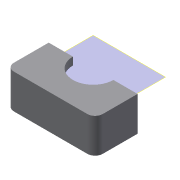
# Autodesk Inventor part: 20_Cube_Insert_Syringepump_Micro_syringeclamp_v3
Saved by Autodesk Inventor 2022 (Build 260153000, 153)
## iProperties
Created: 2022-01-11
Part Number: 20_Cube_Insert_Syringepump_Micro_syringeclamp_v3
Material: Generisch
Document SubType Name: Modeling
Designer: diederichbenedict
Density: 1 g/cm^3
Appearance: Vorgabe
Author: diederichbenedict
Autodesk Inventor part; units mm, degrees
ref_plane "YZ Plane" through (0, 0, 0) normal (1, 0, 0) x (0, 1, 0)
ref_plane "XZ Plane" through (0, 0, 0) normal (0, 1, 0) x (-1, 0, 0)
ref_plane "XY Plane" through (0, 0, 0) normal (0, 0, 1) x (1, 0, 0)
ref_plane "Arbeitsebene1" through (-12.85, 3.6, -4.5) normal (0, -1, 0) x (0, 0, 1)
sketch "Skizze1" plane through (-12.85, 3.6, -4.5) normal (0, -1, 0) x (0, 0, 1)
  circle A0 centre (0, 0) radius 4.3 construction
  line L0 (0.4805, 5.7801) -> (0.4805, 4.5246)
  line L1 (0.4805, -4.5246) -> (0.4805, -5.7801)
  line L2 (0, -5.8) -> (5.55, -5.8)
  line L3 (5.55, -5.8) -> (5.55, 5.8)
  line L4 (5.55, 5.8) -> (0, 5.8)
  line L5 (0, 5.8) -> (0, -5.8)
  line L6 (0, -4.55) -> (4.55, -4.55)
  line L7 (4.55, -4.55) -> (4.55, 4.55)
  line L8 (4.55, 4.55) -> (0, 4.55)
  line L9 (0, 4.55) -> (0, -4.55)
  point P0 (4.5, -12.85)
  point P1 (0, 4.55)
  dimension "d2" = 0
  dimension "d27" = 0
  dimension "d28" = 1
  constraints: 20 end point, 4 parallel, 2 horizontal, 2 perpendicular, 2 vertical, 1 point on line
  measures "d2" distance between parallel lines of L1 L0
  measures "d27" distance from line of A0.centre L5
  measures "d28" distance between parallel lines of L7 L3
extrude "Extrusion1" add sketch "Skizze1" along normal blind 2.5 contours L5 L6 L7 L8 L4 L3 L2
sketch "Skizze2" plane through (-12.85, 1.1, -4.5) normal (0, -1, 0) x (1, 0, 0)
  line L0 (-5.7801, 0.4805) -> (5.7801, 0.4805)
  line L1 (-5.8, 0) -> (-4.55, 0) projected
  line L2 (-4.55, 0) -> (-4.55, 4.55) projected
  line L3 (-4.55, 4.55) -> (4.55, 4.55) projected
  line L4 (4.55, 4.55) -> (4.55, 0) projected
  line L5 (4.55, 0) -> (5.8, 0) projected
  line L6 (5.8, 0) -> (5.8, 5.55) projected
  line L7 (5.8, 5.55) -> (-5.8, 5.55) projected
  line L8 (-5.8, 5.55) -> (-5.8, 0) projected
  line L9 (-4.55, 0) -> (4.55, 0)
  point P0 (12.85, 4.5)
  constraints: 4 end point, 2 horizontal
extrude "Extrusion2" add sketch "Skizze2" along normal blind 1
sketch "Skizze7" plane through (-12.85, 3.6, -4.5) normal (0, 1, 0) x (1, 0, 0)
  line L0 (-5.8, 0) -> (-4.55, 0) projected
  line L1 (-5.8, -5.55) -> (-5.8, 0) projected
  line L2 (5.8, -5.55) -> (-5.8, -5.55) projected
  line L3 (5.8, 0) -> (5.8, -5.55) projected
  line L4 (4.55, 0) -> (5.8, 0) projected
  line L5 (4.55, -4.55) -> (4.55, 0) projected
  line L6 (-4.55, -4.55) -> (4.55, -4.55) projected
  line L7 (-4.55, 0) -> (-4.55, -4.55) projected
  line L8 (4.55, 0) -> (-4.55, 0)
  line L9 (-4.55, -4.55) -> (4.55, -4.55) projected
  circle A0 centre (0, 0) radius 2.6359
  point P0 (12.85, -4.5)
  point P1 (2.6359, 0)
  point P2 (-2.6359, 0)
  constraints: 2 end point, 1 centre point, 1 midpoint, 1 parallel
extrude "Extrusion6" add sketch "Skizze7" along normal blind 1 contours L0 L7 L6 L5 L4 L3 L2 L1 | L8 A0 L5 L6 L7
fillet "Rundung2" radius 1 2 edges at (-18.65, 2.35, 1.05) (-7.05, 2.35, 1.05)
